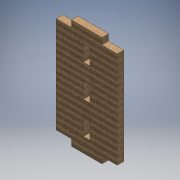
# Autodesk Inventor part: IBeamVertical
Saved by Autodesk Inventor 2016 (Build 200138000, 138)
## iProperties
Created: 2015-12-07
Part Number: IBeamVertical
Material: MDF Medium Density Fiberboard
Document SubType Name: Modeling
Designer: momem
Density: 0.8 g/cm^3
Appearance: Cardboard - Corrugated
d7: 94.601 mm
Author: momem
Autodesk Inventor part; units mm, degrees
ref_plane "YZ Plane" through (0, 0, 0) normal (1, 0, 0) x (0, 1, 0)
ref_plane "XZ Plane" through (0, 0, 0) normal (0, 1, 0) x (-1, 0, 0)
ref_plane "XY Plane" through (0, 0, 0) normal (0, 0, 1) x (1, 0, 0)
sketch "Sketch1" plane through (0, 0, 0) normal (0, 1, 0) x (-1, 0, 0)
  line L0 (44.835, 0) -> (44.835, -6.39)
  line L1 (44.835, -6.39) -> (14.945, -6.39)
  line L2 (14.945, -6.39) -> (14.945, 0)
  line L3 (14.945, 0) -> (0, 0)
  line L4 (44.835, 0) -> (59.78, 0)
  line L5 (59.78, 0) -> (59.78, 94.6011)
  line L6 (0, 0) -> (0, 94.6011)
  line L7 (59.78, 47.3006) -> (0, 47.3006) construction
  line L8 (44.835, 94.6011) -> (44.835, 100.9911)
  line L9 (44.835, 100.9911) -> (14.945, 100.9911)
  line L10 (14.945, 100.9911) -> (14.945, 94.6011)
  line L11 (14.945, 94.6011) -> (0, 94.6011)
  line L12 (44.835, 94.6011) -> (59.78, 94.6011)
  line L13 (29.89, -6.39) -> (29.89, 100.9911) construction
  line L14 (26.727, 23.6503) -> (33.0531, 23.6503)
  line L15 (33.0531, 23.6503) -> (33.0531, 7.8834)
  line L16 (33.0531, 7.8834) -> (26.727, 7.8834)
  line L17 (26.727, 7.8834) -> (26.727, 23.6503)
  line L18 (33.0531, 15.7669) -> (26.727, 15.7669) construction
  line L19 (26.727, 55.184) -> (33.0531, 55.184)
  line L20 (33.0531, 47.3006) -> (26.727, 47.3006) construction
  line L21 (33.0531, 55.184) -> (33.0531, 39.4171)
  line L22 (26.727, 39.4171) -> (26.727, 55.184)
  line L23 (33.0531, 39.4171) -> (26.727, 39.4171)
  line L24 (26.727, 86.7177) -> (33.0531, 86.7177)
  line L25 (33.0531, 78.8343) -> (26.727, 78.8343) construction
  line L26 (33.0531, 86.7177) -> (33.0531, 70.9509)
  line L27 (26.727, 70.9509) -> (26.727, 86.7177)
  line L28 (33.0531, 70.9509) -> (26.727, 70.9509)
  point P0 (29.89, 7.8834)
  point P1 (29.89, 39.4171)
  point P2 (29.89, 70.9509)
  dimension "d0" = 29.89
  dimension "d1" = 14.945
  dimension "d2" = 14.945
  dimension "d3" = 6.39
  dimension "d4" = 15.7669
  dimension "d6" = 6.3261
  dimension "d7" = 94.6011
  dimension "d15" = 7.8834
  dimension "d47" = 31.5337
  constraints: 58 end point, 7 midpoint, 4 perpendicular, 4 symmetric about line, 4 vertical, 3 parallel, 2 horizontal, 1 coincident, 1 collinear, 1 vertical alignment, 24 other
  measures "d0" distance of L0.end L1.end
  measures "d1" distance of L0.start L4.end
  measures "d2" distance of L2.end L3.end
  measures "d3" distance of L0.start L0.end
  measures "d4" distance of L14.end L15.end
  measures "d6" distance of L15.end L16.end
  measures "d7" distance of L4.end L5.end
  measures "d15" distance from line of L4 point (29.89, 7.883)
  measures "d47" distance of L14.start L19.start
extrude "Extrusion4" add sketch "Sketch1" along normal blind 6.39
equation "\"d0\" = 0.5 * ColumnWidth"
equation "\"d1\" = 0.25 * ColumnWidth"
equation "\"d2\" = 0.25 * ColumnWidth"
equation "\"d3\" = WoodThickness"
equation "\"d4\" = 0.166667 * d7"
equation "\"d6\" = 0.99 * WoodThickness"
equation "\"d15\" = 0.0833333 * d7"
equation "\"d47\" = 0.333333 * d7"
equation "\"d52\" = WoodThickness"
equation "\"ColumnWidth\" = 59.78"
equation "\"WoodThickness\" = 6.39"
body "Solid4"
